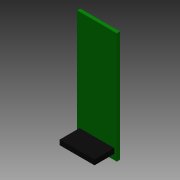
# Autodesk Inventor part: Sensor_Board_dummy
Saved by Autodesk Inventor 2016 (Build 200138000, 138)
## iProperties
Created: 2014-12-25
Part Number: Sensor_Board_dummy
Material: Generic
Document SubType Name: Modeling
Designer: Openlab
Density: 1 g/cm^3
Appearance: Dark Green
Mass: 2.2704 g
Surface Area: 29.3619 cm^2
Volume: 2.2704 cm^3
Author: Openlab
Autodesk Inventor part; units mm, degrees
ref_plane "YZ Plane" through (0, 0, 0) normal (1, 0, 0) x (0, 1, 0)
ref_plane "XZ Plane" through (0, 0, 0) normal (0, 1, 0) x (-1, 0, 0)
ref_plane "XY Plane" through (0, 0, 0) normal (0, 0, 1) x (1, 0, 0)
sketch "Sketch2" plane through (0, 0, 0) normal (0, 1, 0) x (-1, 0, 0)
  line L0 (20, 0) -> (0, 0)
  line L1 (0, 0) -> (0, -56)
  line L2 (0, -56) -> (20, -56)
  line L3 (20, -56) -> (20, 0)
  line L4 (18.75, -50.75) -> (1.25, -50.75)
  line L5 (1.25, -50.75) -> (1.25, -53.25)
  line L6 (1.25, -53.25) -> (18.75, -53.25)
  line L7 (18.75, -53.25) -> (18.75, -50.75)
  line L8 (11.9, -6.7) -> (8.1, -6.7)
  line L9 (8.1, -6.7) -> (8.1, -9.3)
  line L10 (8.1, -9.3) -> (11.9, -9.3)
  line L11 (11.9, -9.3) -> (11.9, -6.7)
  line L12 (11.9, -42.7) -> (8.1, -42.7)
  line L13 (8.1, -42.7) -> (8.1, -45.3)
  line L14 (8.1, -45.3) -> (11.9, -45.3)
  line L15 (11.9, -45.3) -> (11.9, -42.7)
  line L16 (8.1, -27.3) -> (11.9, -27.3)
  line L17 (8.1, -24.7) -> (8.1, -27.3)
  line L18 (11.9, -24.7) -> (8.1, -24.7)
  line L19 (11.9, -27.3) -> (11.9, -24.7)
  line L20 (23.6892, -52) -> (-2.3247, -52) construction
  line L21 (10, -54.7987) -> (10, -48.1542) construction
  line L22 (10, 9.3713) -> (10, -46.1174) construction
  line L23 (11.7769, -8) -> (1.25, -8) construction
  line L24 (11.7769, -26) -> (1.25, -26) construction
  line L25 (11.7769, -44) -> (1.25, -44) construction
  dimension "d0" = 20
  dimension "d1" = 56
  dimension "d2" = 17.5
  dimension "d3" = 2.5
  dimension "d9" = 3.8
  dimension "d10" = 2.6
  dimension "d13" = 3.8
  dimension "d14" = 2.6
  dimension "d30" = 3.8
  dimension "d31" = 2.6
  dimension "d40" = 10
  dimension "d41" = 10
  dimension "d45" = 8.1
  dimension "d46" = 8
  dimension "d47" = 18
  dimension "d48" = 18
  dimension "d49" = 4
  constraints: 52 end point, 10 parallel, 9 horizontal, 5 perpendicular, 2 collinear, 2 vertical, 1 coincident, 7 other
  measures "d0" distance of L2.end L1.end
  measures "d1" distance of L1.end L0.end
  measures "d2" distance of L6.end L5.end
  measures "d3" distance of L5.end L4.end
  measures "d9" distance of L9.end L10.end
  measures "d10" distance of L8.end L9.end
  measures "d13" distance of L14.start L14.end
  measures "d14" distance of L13.start L14.start
  measures "d30" distance of L17.end L19.start
  measures "d31" distance of L18.end L17.end
  measures "d40" distance between parallel lines of L3 L21
  measures "d41" distance between parallel lines of L1 L22
  measures "d45" distance between parallel lines of L1 L9
  measures "d46" distance between parallel lines of L23 L0
  measures "d47" distance between parallel lines of L24 L23
  measures "d48" distance between parallel lines of L25 L24
  measures "d49" distance between parallel lines of L2 L20
extrude "Extrusion1" add sketch "Sketch2" along normal blind 1.6 contours L3 L2 L1 L0 | L7 L6 L5 L4 | L11 L10 L9 L8 | L15 L14 L13 L12 | L17 L18 L19 L16
extrude "Extrusion3" add sketch "Sketch2" against normal blind 10 contours L7 L6 L5 L4
extrude "Extrusion4" add sketch "Sketch2" along normal blind 2.98 contours L11 L10 L9 L8 | L15 L14 L13 L12 | L17 L18 L19 L16
body "Solid1"
